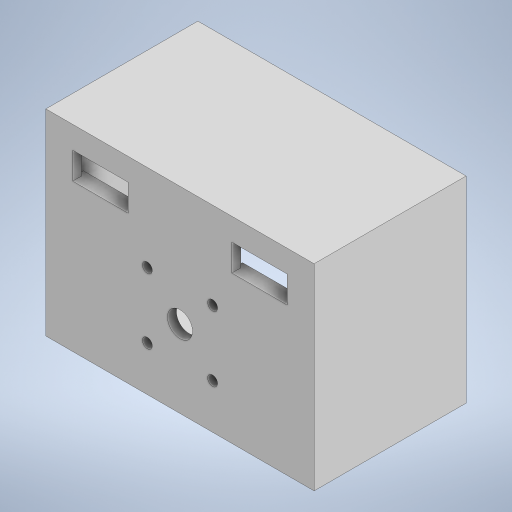
# Autodesk Inventor part: case_1
Saved by Autodesk Inventor 2024 (Build 280153000, 153)
## iProperties
Created: 2026-02-20
Part Number: case_1
Material: Generic
Document SubType Name: Modeling
Designer: janst
Density: 1 g/cm^3
Appearance: Default
Author: janst
## iProperties of the stored document case_1_3DPrint.ipt
Created: 2026-02-20
Part Number: case_1_3DPrint
Material: Generic
Document SubType Name: Modeling
Designer: janst
Density: 1 g/cm^3
Appearance: Default
Author: janst
Autodesk Inventor part; units mm, degrees
ref_plane "YZ Plane" through (0, 0, 0) normal (1, 0, 0) x (0, 1, 0)
ref_plane "XZ Plane" through (0, 0, 0) normal (0, 1, 0) x (-1, 0, 0)
ref_plane "XY Plane" through (0, 0, 0) normal (0, 0, 1) x (1, 0, 0)
sketch "Sketch1" plane through (0, 0, 0) normal (0, 0, 1) x (1, 0, 0)
  line L0 (75, -55) -> (-75, -55)
  line L1 (-75, -55) -> (-75, 55)
  line L2 (-75, 55) -> (75, 55)
  line L3 (75, 55) -> (75, -55)
  line L4 (75, -55) -> (-75, 55) construction
  line L5 (-75, -55) -> (75, 55) construction
  line L6 (18.25, -30) -> (-18.25, -30)
  line L7 (-18.25, -30) -> (-18.25, 6.5)
  line L8 (-18.25, 6.5) -> (18.25, 6.5)
  line L9 (18.25, 6.5) -> (18.25, -30)
  line L10 (18.25, -30) -> (-18.25, 6.5) construction
  line L11 (-18.25, -30) -> (18.25, 6.5) construction
  line L12 (0, -77) -> (0, 77) projected
  line L13 (-29, 27.5) -> (-60, 27.5)
  line L14 (-60, 27.5) -> (-60, 42.5)
  line L15 (-60, 42.5) -> (-29, 42.5)
  line L16 (-29, 42.5) -> (-29, 27.5)
  line L17 (-29, 27.5) -> (-60, 42.5) construction
  line L18 (-60, 27.5) -> (-29, 42.5) construction
  circle A0 centre (0, -11.75) radius 7
  line L19 (60, 27.5) -> (29, 27.5)
  line L20 (29, 27.5) -> (29, 42.5)
  line L21 (29, 42.5) -> (60, 42.5)
  line L22 (60, 42.5) -> (60, 27.5)
  line L23 (60, 27.5) -> (29, 42.5) construction
  line L24 (29, 27.5) -> (60, 42.5) construction
  line L25 (-75, 35) -> (75, 35)
  point P0 (0, 0)
  point P1 (0, -11.75)
  point P2 (-44.5, 35)
  point P3 (44.5, 35)
  dimension "d0" = 110
  dimension "d1" = 150
  dimension "d2" = 36.5
  dimension "d3" = 36.5
  dimension "d4" = 25
  dimension "d5" = 14
  dimension "d6" = 31
  dimension "d7" = 15
  dimension "d8" = 15
  dimension "d9" = 31
  dimension "d11" = 20
  dimension "d12" = 15
  dimension "d13" = 15
  constraints: 50 end point, 9 parallel, 8 midpoint, 5 coincident, 5 point on line, 4 horizontal, 4 perpendicular, 1 centre point
  measures "d0" distance of L2.end L0.start
  measures "d1" distance of L1.end L2.end
  measures "d2" distance of L8.end L6.start
  measures "d3" distance of L6.start L6.end
  measures "d4" distance between parallel lines of L0 L6
  measures "d5" diameter of A0
  measures "d6" distance of L13.start L13.end
  measures "d7" distance of L15.end L13.start
  measures "d8" distance of L19.end L20.end
  measures "d9" distance of L19.start L19.end
  measures "d11" distance between parallel lines of L2 L25
  measures "d12" distance between parallel lines of L1 L14
  measures "d13" distance between parallel lines of L3 L22
extrude "Extrusion1" add sketch "Sketch1" against normal blind 5
extrude "Extrusion2" cut sketch "Sketch1" against normal blind 5 contours L25 L20 L21 L22 | L22 L19 L20 L25 | A0 L12 | L12 A0 | L25 L16 L13 L14 | L14 L15 L16 L25
hole "Hole1" at (-18.25, 6.5, 0) at (-18.25, -30, 0) at (18.25, -30, 0) at (18.25, 6.5, 0) direction (0, 0, -1) diameter 5.5 end through all
sketch "Sketch2" plane through (0, 0, -5) normal (0, 0, -1) x (-1, 0, 0)
  circle A0 centre (-18.25, 6.5) radius 2.75 projected
  circle A1 centre (-18.25, -30) radius 2.75 projected
  circle A2 centre (18.25, -30) radius 2.75 projected
  circle A3 centre (18.25, 6.5) radius 2.75 projected
  circle A4 centre (0, -11.75) radius 7 projected
  line L0 (-29, 27.5) -> (-60, 27.5) projected
  line L1 (-60, 27.5) -> (-60, 42.5) projected
  line L2 (-60, 42.5) -> (-29, 42.5) projected
  line L3 (-29, 42.5) -> (-29, 27.5) projected
  line L4 (29, 42.5) -> (60, 42.5) projected
  line L5 (60, 42.5) -> (60, 27.5) projected
  line L6 (60, 27.5) -> (29, 27.5) projected
  line L7 (29, 27.5) -> (29, 42.5) projected
  line L8 (75, 55) -> (-75, 55) projected
  line L9 (-75, 55) -> (-75, -55) projected
  line L10 (-75, -55) -> (75, -55) projected
  line L11 (75, -55) -> (75, 55) projected
  line L12 (-27, 44.5) -> (-62, 44.5)
  line L13 (-62, 44.5) -> (-62, 25.5)
  line L14 (-62, 25.5) -> (-27, 25.5)
  line L15 (-27, 25.5) -> (-27, 44.5)
  line L16 (62, 44.5) -> (27, 44.5)
  line L17 (27, 44.5) -> (27, 25.5)
  line L18 (27, 25.5) -> (62, 25.5)
  line L19 (62, 25.5) -> (62, 44.5)
  line L20 (-62, 42.5) -> (-27, 42.5)
  line L21 (-62, 27.5) -> (-27, 27.5)
  line L22 (27, 42.5) -> (62, 42.5)
  line L23 (62, 27.5) -> (27, 27.5)
  line L24 (-60, 42.5) -> (-29, 42.5) projected
  line L25 (-29, 27.5) -> (-60, 27.5) projected
  line L26 (29, 42.5) -> (60, 42.5) projected
  point P0 (0, 0)
  dimension "d25" = 2
  dimension "d26" = 2
  constraints: 24 end point, 9 point on line, 3 collinear, 3 parallel, 1 perpendicular, 6 other
  measures "d25" distance between parallel lines of L15 L3
  measures "d26" distance between parallel lines of L17 L7
extrude "Extrusion3" add sketch "Sketch2" along normal blind 3 contours L21 L15 L14 L13 L0 | L2 L20 L13 L12 L15 | L22 L17 L16 L19 L4 | L6 L23 L19 L18 L17
sketch "Sketch3" plane through (0, 0, -5) normal (0, 0, -1) x (-1, 0, 0)
  line L0 (75, 55) -> (-75, 55) projected
  line L1 (-75, 55) -> (-75, -55) projected
  line L2 (-75, -55) -> (75, -55) projected
  line L3 (75, -55) -> (75, 55) projected
  line L4 (-70, 50) -> (70, 50)
  line L5 (70, 50) -> (70, -50)
  line L6 (70, -50) -> (-70, -50)
  line L7 (-70, -50) -> (-70, 50)
  point P0 (0, 0)
  dimension "d29" = 5
  constraints: 8 end point, 3 other
  measures "d29" distance between parallel lines of L0 L4
extrude "Extrusion4" add sketch "Sketch3" along normal blind 80
equation "\"d3\" = d2"
equation "\"d8\" = d7"
equation "\"d9\" = d6"
equation "\"d13\" = d12"
equation "\"d26\" = d25"
body "Solid1"
